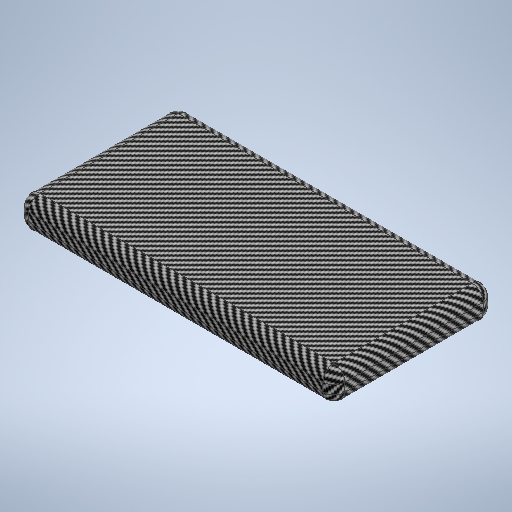
# Autodesk Inventor part: powerbank
Saved by Autodesk Inventor 2025 (Build 290162000, 162)
## iProperties
Created: 2024-09-26
Part Number: powerbank
Material: CFRP
Document SubType Name: Modeling
Designer: DANIEL
Density: 1.43 g/cm^3
Appearance: Carbon Fiber
Author: DANIEL
Autodesk Inventor part; units mm, degrees
ref_plane "YZ Plane" through (0, 0, 0) normal (1, 0, 0) x (0, 1, 0)
ref_plane "XZ Plane" through (0, 0, 0) normal (0, 1, 0) x (-1, 0, 0)
ref_plane "XY Plane" through (0, 0, 0) normal (0, 0, 1) x (1, 0, 0)
sketch "Sketch1" plane through (0, 0, 0) normal (0, 1, 0) x (-1, 0, 0)
  line L0 (72, -36.5) -> (-72, -36.5)
  line L1 (-72, -36.5) -> (-72, 36.5)
  line L2 (-72, 36.5) -> (72, 36.5)
  line L3 (72, 36.5) -> (72, -36.5)
  line L4 (72, -36.5) -> (-72, 36.5) construction
  line L5 (-72, -36.5) -> (72, 36.5) construction
  point P0 (0, 0)
  dimension "d0" = 144
  dimension "d1" = 73
  constraints: 12 end point, 2 midpoint, 2 parallel, 1 horizontal, 1 perpendicular
  measures "d0" distance of L1.end L2.end
  measures "d1" distance of L0.end L1.end
extrude "Extrusion1" add sketch "Sketch1" along normal blind 14
fillet "Fillet1" radius 5 12 edges at (72, 14, 0) (0, 14, 36.5) (0, 14, -36.5) (-72, 14, 0) (0, 0, 36.5) (72, 7, 36.5) (72, 0, 0) (72, 7, -36.5) (0, 0, -36.5) (-72, 0, 0) (-72, 7, -36.5) (-72, 7, 36.5)
body "Solid1"
